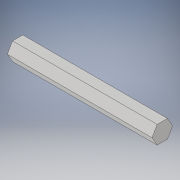
# Autodesk Inventor part: Axle
Saved by Autodesk Inventor 2017 (Build 210142000, 142)
## iProperties
Created: 2017-01-16
Part Number: Axle
Material: Generic
Document SubType Name: Modeling
Designer: mmarkle
Density: 1 g/cm^3
Appearance: Default
Author: mmarkle
Autodesk Inventor part; units mm, degrees
ref_plane "YZ Plane" through (0, 0, 0) normal (1, 0, 0) x (0, 1, 0)
ref_plane "XZ Plane" through (0, 0, 0) normal (0, 1, 0) x (-1, 0, 0)
ref_plane "XY Plane" through (0, 0, 0) normal (0, 0, 1) x (1, 0, 0)
sketch "Sketch1" plane through (0, 0, 0) normal (1, 0, 0) x (0, 1, 0)
  line L0 (10.9985, -6.35) -> (0, -12.7)
  line L1 (0, -12.7) -> (-10.9985, -6.35)
  line L2 (-10.9985, -6.35) -> (-10.9985, 6.35)
  line L3 (-10.9985, 6.35) -> (0, 12.7)
  line L4 (0, 12.7) -> (10.9985, 6.35)
  line L5 (10.9985, 6.35) -> (10.9985, -6.35)
  point P0 (0, 0)
  point P1 (0, 0)
  dimension "d0" = 12.7
  constraints: 12 end point, 1 coincident, 13 other
  measures "d0" distance of L4.end L0.start
extrude "Extrusion1" add sketch "Sketch1" along normal blind 177.8
body "Solid1"
